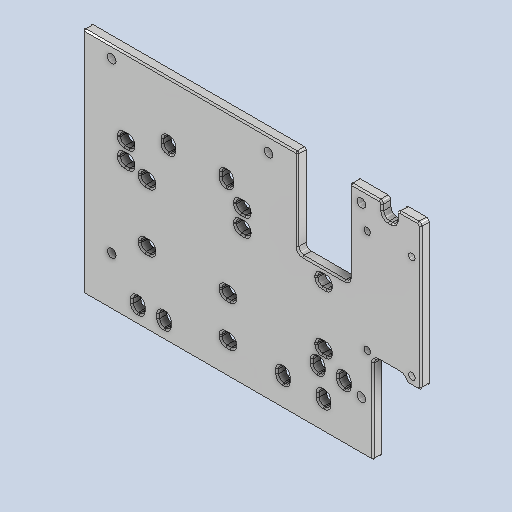
# Autodesk Inventor part: Cable_Fastener_WaveRunner
Saved by Autodesk Inventor 2022 (Build 260153000, 153)
## iProperties
Created: 2020-06-16
Part Number: Cable_Fastener_WaveRunner
Material: Generic
Document SubType Name: Modeling
Designer: Viktor Lindström
Density: 1 g/cm^3
Appearance: Default
Author: Viktor Lindström
Autodesk Inventor part; units mm, degrees
ref_plane "YZ Plane" through (0, 0, 0) normal (1, 0, 0) x (0, 1, 0)
ref_plane "XZ Plane" through (0, 0, 0) normal (0, 1, 0) x (-1, 0, 0)
ref_plane "XY Plane" through (0, 0, 0) normal (0, 0, 1) x (1, 0, 0)
sketch "Sketch1" plane through (0, 0, 0) normal (0, 0, 1) x (1, 0, 0)
  line L0 (-50, -39.5) -> (50, -39.5)
  line L1 (50, -39.5) -> (50, 39.5)
  line L2 (50, 39.5) -> (-50, 39.5)
  line L3 (-50, 39.5) -> (-50, -39.5)
  line L4 (-50, -39.5) -> (50, 39.5) construction
  line L5 (50, -39.5) -> (-50, 39.5) construction
  point P0 (0, 0)
  dimension "d0" = 100
  dimension "d1" = 79
  constraints: 12 end point, 2 midpoint, 2 parallel, 1 horizontal, 1 perpendicular
  measures "d0" distance of L1.end L2.end
  measures "d1" distance of L0.end L1.end
extrude "Extrusion1" add sketch "Sketch1" along normal blind 3
sketch "Sketch2" plane through (0, 0, 3) normal (0, 0, 1) x (1, 0, 0)
  circle A0 centre (-40, 35.5) radius 1.5
  circle A1 centre (46, 35.5) radius 1.5
  line L0 (50, 39.5) -> (-50, 39.5) projected
  line L1 (50, -39.5) -> (50, 39.5) projected
  line L2 (-73.7236, 6.5) -> (70.0965, 6.5) construction
  circle A2 centre (-40, -22.5) radius 1.5
  circle A3 centre (46, -22.5) radius 1.5
  point P0 (0, 0)
  dimension "d4" = 3
  dimension "d5" = 3
  dimension "d6" = 86
  dimension "d7" = 4
  dimension "d8" = 4
  dimension "d9" = 4
  dimension "d10" = 33
  constraints: 4 centre point, 2 end point, 2 symmetric about line, 1 horizontal, 2 other
  measures "d4" diameter of A0
  measures "d5" diameter of A1
  measures "d6" distance of A1.centre A0.centre
  measures "d7" distance from line of L0 A1.centre
  measures "d8" distance from line of L0 A0.centre
  measures "d9" distance from line of L1 A1.centre
  measures "d10" distance between parallel lines of L0 L2
extrude "Extrusion2" cut sketch "Sketch2" against normal through all
fillet "Fillet1" radius 0.6 3 edges at (-50, 39.5, 1.5) (-50, -39.5, 1.5) (50, -39.5, 1.5)
sketch "Sketch3" plane through (0, 0, 3) normal (0, 0, 1) x (1, 0, 0)
  line L0 (31, -32) -> (35, -32)
  line L1 (35, -32) -> (35, -27)
  line L2 (35, -27) -> (31, -27)
  line L3 (31, -27) -> (31, -32)
  line L4 (31, -32) -> (35, -27) construction
  line L5 (35, -32) -> (31, -27) construction
  line L6 (21, -27) -> (17, -27)
  line L7 (17, -27) -> (17, -32)
  line L8 (17, -32) -> (21, -32)
  line L9 (21, -32) -> (21, -27)
  line L10 (21, -27) -> (17, -32) construction
  line L11 (17, -27) -> (21, -32) construction
  line L12 (-2.5, -30.5) -> (2.5, -30.5)
  line L13 (2.5, -30.5) -> (2.5, -26.5)
  line L14 (2.5, -26.5) -> (-2.5, -26.5)
  line L15 (-2.5, -26.5) -> (-2.5, -30.5)
  line L16 (-2.5, -30.5) -> (2.5, -26.5) construction
  line L17 (2.5, -30.5) -> (-2.5, -26.5) construction
  line L18 (-2.5, -12.5) -> (2.5, -12.5)
  line L19 (2.5, -12.5) -> (2.5, -16.5)
  line L20 (2.5, -16.5) -> (-2.5, -16.5)
  line L21 (-2.5, -16.5) -> (-2.5, -12.5)
  line L22 (-2.5, -12.5) -> (2.5, -16.5) construction
  line L23 (2.5, -12.5) -> (-2.5, -16.5) construction
  line L24 (-18.5, 17) -> (-22.5, 17)
  line L25 (-22.5, 17) -> (-22.5, 22)
  line L26 (-22.5, 22) -> (-18.5, 22)
  line L27 (-18.5, 22) -> (-18.5, 17)
  line L28 (-18.5, 17) -> (-22.5, 22) construction
  line L29 (-22.5, 17) -> (-18.5, 22) construction
  line L30 (1.5, 17) -> (-2.5, 17)
  line L31 (-2.5, 17) -> (-2.5, 22)
  line L32 (-2.5, 22) -> (1.5, 22)
  line L33 (1.5, 22) -> (1.5, 17)
  line L34 (1.5, 17) -> (-2.5, 22) construction
  line L35 (-2.5, 17) -> (1.5, 22) construction
  line L36 (30.5, 3.5) -> (35.5, 3.5)
  line L37 (35.5, 3.5) -> (35.5, 7.5)
  line L38 (35.5, 7.5) -> (30.5, 7.5)
  line L39 (30.5, 7.5) -> (30.5, 3.5)
  line L40 (30.5, 3.5) -> (35.5, 7.5) construction
  line L41 (35.5, 3.5) -> (30.5, 7.5) construction
  line L42 (-30.3047, -16.5) -> (-25.3047, -16.5)
  line L43 (-25.3047, -16.5) -> (-25.3047, -12.5)
  line L44 (-25.3047, -12.5) -> (-30.3047, -12.5)
  line L45 (-30.3047, -12.5) -> (-30.3047, -16.5)
  line L46 (-30.3047, -16.5) -> (-25.3047, -12.5) construction
  line L47 (-25.3047, -16.5) -> (-30.3047, -12.5) construction
  line L48 (-25.3047, 3.5) -> (-30.3047, 3.5)
  line L49 (-30.3047, 3.5) -> (-30.3047, 7.5)
  line L50 (-30.3047, 7.5) -> (-25.3047, 7.5)
  line L51 (-25.3047, 7.5) -> (-25.3047, 3.5)
  line L52 (-25.3047, 3.5) -> (-30.3047, 7.5) construction
  line L53 (-30.3047, 3.5) -> (-25.3047, 7.5) construction
  line L54 (50, -38.9) -> (50, 39.5) projected
  line L55 (-49.4, -39.5) -> (49.4, -39.5) projected
  line L56 (50, 39.5) -> (-49.4, 39.5) projected
  line L57 (35.5, -16.5) -> (30.5, -16.5)
  line L58 (30.5, -16.5) -> (30.5, -12.5)
  line L59 (30.5, -12.5) -> (35.5, -12.5)
  line L60 (35.5, -12.5) -> (35.5, -16.5)
  line L61 (35.5, -16.5) -> (30.5, -12.5) construction
  line L62 (30.5, -16.5) -> (35.5, -12.5) construction
  line L63 (-50, 38.9) -> (-50, -38.9) projected
  point P0 (0, 0)
  point P1 (33, -29.5)
  point P2 (19, -29.5)
  point P3 (0, -28.5)
  point P4 (0, -14.5)
  point P5 (-20.5, 19.5)
  point P6 (-0.5, 19.5)
  point P7 (33, 5.5)
  point P8 (-27.8047, -14.5)
  point P9 (-27.8047, 5.5)
  point P10 (50, 38.9)
  point P11 (49.4, 39.5)
  point P12 (33, -14.5)
  dimension "d14" = 4
  dimension "d15" = 4
  dimension "d16" = 4
  dimension "d17" = 4
  dimension "d18" = 4
  dimension "d19" = 4
  dimension "d20" = 4
  dimension "d21" = 4
  dimension "d23" = 4
  dimension "d24" = 5
  dimension "d25" = 5
  dimension "d26" = 5
  dimension "d27" = 5
  dimension "d29" = 5
  dimension "d30" = 5
  dimension "d31" = 5
  dimension "d32" = 5
  dimension "d33" = 5
  dimension "d34" = 0
  dimension "d35" = 20
  dimension "d36" = 20
  dimension "d37" = 14
  dimension "d38" = 14
  dimension "d40" = 17
  dimension "d41" = 10
  dimension "d42" = 25
  dimension "d43" = 50
  dimension "d44" = 34
  dimension "d45" = 4
  dimension "d46" = 5
  dimension "d47" = 20
  dimension "d48" = 0
  dimension "d49" = 0
  dimension "d50" = 17
  dimension "d125" = 20
  dimension "d126" = 29.5
  constraints: 120 end point, 20 midpoint, 20 parallel, 10 horizontal, 10 perpendicular, 3 point on line
  measures "d14" distance of L14.end L12.start
  measures "d15" distance of L18.end L19.end
  measures "d16" distance of L44.end L42.start
  measures "d17" distance of L48.end L49.end
  measures "d18" distance of L24.start L24.end
  measures "d19" distance of L30.start L30.end
  measures "d20" distance of L6.start L6.end
  measures "d21" distance of L1.end L2.end
  measures "d23" distance of L38.end L36.start
  measures "d24" distance of L12.start L12.end
  measures "d25" distance of L19.end L20.end
  measures "d26" distance of L6.end L7.end
  measures "d27" distance of L2.end L0.start
  measures "d29" distance of L36.start L36.end
  measures "d30" distance of L32.end L30.start
  measures "d31" distance of L26.end L24.start
  measures "d32" distance of L48.start L48.end
  measures "d33" distance of L42.start L42.end
  measures "d34" vertical distance of point (33, -29.5) point (19, -29.5)
  measures "d35" distance of point (-27.805, 5.5) point (-27.805, -14.5)
  measures "d36" distance of point (-0.5, 19.5) point (-20.5, 19.5)
  measures "d37" distance of point (33, -29.5) point (19, -29.5)
  measures "d38" distance of point (0, -14.5) point (0, -28.5)
  measures "d40" distance from line of L54 point (33, -29.5)
  measures "d41" distance from line of L55 point (33, -29.5)
  measures "d42" distance from line of L55 point (0, -14.5)
  measures "d43" distance from line of L54 point (0, -28.5)
  measures "d44" distance from line of L56 point (-27.805, 5.5)
  measures "d45" distance of L57.end L58.end
  measures "d46" distance of L58.end L59.end
  measures "d47" distance of point (33, 5.5) point (33, -14.5)
  measures "d48" horizontal distance of point (33, 5.5) point (33, -14.5)
  measures "d49" vertical distance of point (33, -14.5) point (-27.805, -14.5)
  measures "d50" distance from line of L54 point (33, -14.5)
  measures "d125" distance from line of L56 point (-20.5, 19.5)
  measures "d126" distance from line of L63 point (-20.5, 19.5)
extrude "Extrusion3" cut sketch "Sketch3" against normal through all
sketch "Sketch4" plane through (0, 0, 3) normal (0, 0, 1) x (1, 0, 0)
  line L0 (-29, -36) -> (-33, -36)
  line L1 (-33, -36) -> (-33, -31)
  line L2 (-33, -31) -> (-29, -31)
  line L3 (-29, -31) -> (-29, -36)
  line L4 (-29, -36) -> (-33, -31) construction
  line L5 (-33, -36) -> (-29, -31) construction
  line L6 (-25.3047, -16.5) -> (-30.3047, -16.5) projected
  line L7 (-30.3047, -12.5) -> (-25.3047, -12.5) projected
  line L8 (-20, -36) -> (-24, -36)
  line L9 (-24, -36) -> (-24, -31)
  line L10 (-24, -31) -> (-20, -31)
  line L11 (-20, -31) -> (-20, -36)
  line L12 (-20, -36) -> (-24, -31) construction
  line L13 (-24, -36) -> (-20, -31) construction
  line L14 (-50, 38.9) -> (-50, -38.9) projected
  line L15 (-49.4, -39.5) -> (49.4, -39.5) projected
  line L16 (32.9777, -23) -> (28.9777, -23)
  line L17 (28.9777, -23) -> (28.9777, -18)
  line L18 (28.9777, -18) -> (32.9777, -18)
  line L19 (32.9777, -18) -> (32.9777, -23)
  line L20 (32.9777, -23) -> (28.9777, -18) construction
  line L21 (28.9777, -23) -> (32.9777, -18) construction
  line L22 (41.9777, -23) -> (37.9777, -23)
  line L23 (37.9777, -23) -> (37.9777, -18)
  line L24 (37.9777, -18) -> (41.9777, -18)
  line L25 (41.9777, -18) -> (41.9777, -23)
  line L26 (41.9777, -23) -> (37.9777, -18) construction
  line L27 (37.9777, -23) -> (41.9777, -18) construction
  line L28 (50, -38.9) -> (50, 39.5) projected
  line L29 (35, -27) -> (35, -32) projected
  line L30 (31, -27) -> (35, -27) projected
  point P0 (0, 0)
  point P1 (-31, -33.5)
  point P2 (-22, -33.5)
  point P3 (30.9777, -20.5)
  point P4 (39.9777, -20.5)
  point P5 (50, 38.9)
  dimension "d54" = 4
  dimension "d55" = 5
  dimension "d56" = 4
  dimension "d57" = 5
  dimension "d60" = 4
  dimension "d61" = 5
  dimension "d64" = 0
  dimension "d65" = 5
  dimension "d66" = 19
  dimension "d67" = 6
  dimension "d72" = 4
  dimension "d73" = 5
  dimension "d74" = 4
  dimension "d75" = 5
  dimension "d76" = 0
  dimension "d77" = 5
  dimension "d82" = 10.0223
  dimension "d83" = 2.0223
  dimension "d84" = 4
  constraints: 48 end point, 8 midpoint, 8 parallel, 4 horizontal, 4 perpendicular
  measures "d54" distance from line of L7 L6.end
  measures "d55" distance of L6.start L6.end
  measures "d56" distance of L0.start L0.end
  measures "d57" distance of L0.end L1.end
  measures "d60" distance of L8.start L8.end
  measures "d61" distance of L8.end L9.end
  measures "d64" vertical distance of point (-31, -33.5) point (-22, -33.5)
  measures "d65" distance between parallel lines of L3 L9
  measures "d66" distance from line of point (-31, -33.5) L14
  measures "d67" distance from line of L15 point (-31, -33.5)
  measures "d72" distance of L16.start L16.end
  measures "d73" distance of L16.end L17.end
  measures "d74" distance of L25.end L22.end
  measures "d75" distance of L22.end L24.start
  measures "d76" vertical distance of point (30.978, -20.5) point (39.978, -20.5)
  measures "d77" distance between parallel lines of L19 L23
  measures "d82" distance from line of L28 point (39.978, -20.5)
  measures "d83" distance between parallel lines of L29 L19
  measures "d84" distance between parallel lines of L30 L16
extrude "Extrusion4" cut sketch "Sketch4" against normal through all
sketch "Sketch5" plane through (0, 0, 3) normal (0, 0, 1) x (1, 0, 0)
  line L0 (-20, -31) -> (-20, -36) projected
  line L1 (-24, -31) -> (-20, -31) projected
  line L2 (-24, -36) -> (-24, -31) projected
  line L3 (-20, -36) -> (-24, -36) projected
  line L4 (-32.5, 15.5) -> (-37.5, 15.5)
  line L5 (-37.5, 15.5) -> (-37.5, 11.5)
  line L6 (-37.5, 11.5) -> (-32.5, 11.5)
  line L7 (-32.5, 11.5) -> (-32.5, 15.5)
  line L8 (-32.5, 15.5) -> (-37.5, 11.5) construction
  line L9 (-37.5, 15.5) -> (-32.5, 11.5) construction
  line L10 (-37.5, 9.5) -> (-32.5, 9.5)
  line L11 (-32.5, 9.5) -> (-32.5, 5.5)
  line L12 (-32.5, 5.5) -> (-37.5, 5.5)
  line L13 (-37.5, 5.5) -> (-37.5, 9.5)
  line L14 (-37.5, 9.5) -> (-32.5, 5.5) construction
  line L15 (-32.5, 9.5) -> (-37.5, 5.5) construction
  line L16 (50, 39.5) -> (-49.4, 39.5) projected
  line L17 (-50, 38.9) -> (-50, -38.9) projected
  line L18 (7.5, 15.5) -> (2.5, 15.5)
  line L19 (2.5, 15.5) -> (2.5, 11.5)
  line L20 (2.5, 11.5) -> (7.5, 11.5)
  line L21 (7.5, 11.5) -> (7.5, 15.5)
  line L22 (7.5, 15.5) -> (2.5, 11.5) construction
  line L23 (2.5, 15.5) -> (7.5, 11.5) construction
  line L24 (2.5, 9.5) -> (7.5, 9.5)
  line L25 (7.5, 9.5) -> (7.5, 5.5)
  line L26 (7.5, 5.5) -> (2.5, 5.5)
  line L27 (2.5, 5.5) -> (2.5, 9.5)
  line L28 (2.5, 9.5) -> (7.5, 5.5) construction
  line L29 (7.5, 9.5) -> (2.5, 5.5) construction
  line L30 (50, -38.9) -> (50, 39.5) projected
  point P0 (-35, 13.5)
  point P1 (-35, 7.5)
  point P2 (49.4, 39.5)
  point P3 (5, 13.5)
  point P4 (5, 7.5)
  point P5 (50, 38.9)
  dimension "d87" = 5
  dimension "d88" = 4
  dimension "d89" = 4
  dimension "d90" = 4
  dimension "d91" = 5
  dimension "d92" = 5
  dimension "d93" = 6
  dimension "d102" = 26
  dimension "d103" = 15
  dimension "d105" = 4
  dimension "d106" = 4
  dimension "d107" = 5
  dimension "d108" = 5
  dimension "d109" = 6
  dimension "d121" = 0
  dimension "d122" = 45
  constraints: 48 end point, 8 midpoint, 8 parallel, 4 horizontal, 4 perpendicular, 2 point on line
  measures "d87" distance of L0.start L0.end
  measures "d88" distance of L1.start L0.start
  measures "d89" distance between parallel lines of L12 L10
  measures "d90" distance of L4.end L5.end
  measures "d91" distance of L10.start L10.end
  measures "d92" distance of L5.end L6.end
  measures "d93" distance of point (-35, 7.5) point (-35, 13.5)
  measures "d102" distance from line of L16 point (-35, 13.5)
  measures "d103" distance from line of L17 point (-35, 13.5)
  measures "d105" distance between parallel lines of L26 L24
  measures "d106" distance of L18.end L19.end
  measures "d107" distance of L24.start L24.end
  measures "d108" distance of L19.end L20.end
  measures "d109" distance of point (5, 7.5) point (5, 13.5)
  measures "d121" distance between parallel lines of L4 L18
  measures "d122" distance from line of L30 point (5, 13.5)
extrude "Extrusion5" cut sketch "Sketch5" against normal through all contours L7 L6 L5 L4 | L10 L11 L12 L13 | L21 L20 L19 L18 | L24 L25 L26 L27
sketch "Sketch6" plane through (0, 0, 3) normal (0, 0, 1) x (1, 0, 0)
  line L0 (50, 39.5) -> (-49.4, 39.5) projected
  line L1 (24, 39.5) -> (42, 39.5)
  line L2 (42, 39.5) -> (42, 9.5)
  line L3 (42, 9.5) -> (24, 9.5)
  line L4 (24, 9.5) -> (24, 39.5)
  line L5 (50, -38.9) -> (50, 39.5) projected
  point P0 (0, 0)
  point P1 (49.4, 39.5)
  point P2 (50, 38.9)
  dimension "d127" = 30
  dimension "d128" = 8
  dimension "d129" = 18
  constraints: 8 end point, 2 parallel, 1 horizontal, 1 perpendicular, 1 point on line
  measures "d127" distance between parallel lines of L0 L3
  measures "d128" distance between parallel lines of L5 L2
  measures "d129" distance between parallel lines of L2 L4
extrude "Extrusion6" cut sketch "Sketch6" against normal through all
fillet "Fillet2" radius 0.6 2 edges at (24, 39.5, 1.5) (42, 39.5, 1.5)
fillet "Fillet2" radius 1.75 2 edges at (42, 9.5, 1.5) (24, 9.5, 1.5)
sketch "Sketch7" plane through (0, 0, 3) normal (0, 0, 1) x (1, 0, 0)
  circle A0 centre (-40, -22.5) radius 1.5 projected
  circle A1 centre (-40, 35.5) radius 1.5 projected
  circle A2 centre (46, -22.5) radius 1.5 projected
  circle A3 centre (46, 35.5) radius 1.5 projected
  arc A4 (42.6, 39.5) -> (42, 38.9) centre (42.6, 38.9) ccw projected
  line L0 (42, 38.9) -> (42, 11.25) projected
  line L1 (40.25, 9.5) -> (25.75, 9.5) projected
  line L2 (24, 11.25) -> (24, 38.9) projected
  arc A5 (24, 38.9) -> (23.4, 39.5) centre (23.4, 38.9) ccw projected
  line L3 (23.4, 39.5) -> (-49.4, 39.5) projected
  arc A6 (-49.4, 39.5) -> (-50, 38.9) centre (-49.4, 38.9) ccw projected
  line L4 (-50, 38.9) -> (-50, -38.9) projected
  arc A7 (-50, -38.9) -> (-49.4, -39.5) centre (-49.4, -38.9) ccw projected
  line L5 (-49.4, -39.5) -> (49.4, -39.5) projected
  arc A8 (49.4, -39.5) -> (50, -38.9) centre (49.4, -38.9) ccw projected
  line L6 (50, -38.9) -> (50, 39.5) projected
  line L7 (50, 39.5) -> (42.6, 39.5) projected
  line L8 (-30.3047, -12.5) -> (-25.3047, -12.5) projected
  line L9 (-25.3047, -12.5) -> (-25.3047, -16.5) projected
  line L10 (-25.3047, -16.5) -> (-30.3047, -16.5) projected
  line L11 (-30.3047, -16.5) -> (-30.3047, -12.5) projected
  line L12 (2.5, -12.5) -> (2.5, -16.5) projected
  line L13 (2.5, -16.5) -> (-2.5, -16.5) projected
  line L14 (-2.5, -16.5) -> (-2.5, -12.5) projected
  line L15 (-2.5, -12.5) -> (2.5, -12.5) projected
  line L16 (30.5, -16.5) -> (30.5, -12.5) projected
  line L17 (30.5, -12.5) -> (35.5, -12.5) projected
  line L18 (35.5, -12.5) -> (35.5, -16.5) projected
  line L19 (35.5, -16.5) -> (30.5, -16.5) projected
  line L20 (31, -27) -> (35, -27) projected
  line L21 (35, -27) -> (35, -32) projected
  line L22 (35, -32) -> (31, -32) projected
  line L23 (31, -32) -> (31, -27) projected
  line L24 (-2.5, 17) -> (-2.5, 22) projected
  line L25 (-2.5, 22) -> (1.5, 22) projected
  line L26 (1.5, 22) -> (1.5, 17) projected
  line L27 (1.5, 17) -> (-2.5, 17) projected
  line L28 (-30.3047, 3.5) -> (-30.3047, 7.5) projected
  line L29 (-30.3047, 7.5) -> (-25.3047, 7.5) projected
  line L30 (-25.3047, 7.5) -> (-25.3047, 3.5) projected
  line L31 (-25.3047, 3.5) -> (-30.3047, 3.5) projected
  line L32 (-2.5, -26.5) -> (2.5, -26.5) projected
  line L33 (2.5, -26.5) -> (2.5, -30.5) projected
  line L34 (2.5, -30.5) -> (-2.5, -30.5) projected
  line L35 (-2.5, -30.5) -> (-2.5, -26.5) projected
  line L36 (30.5, 7.5) -> (35.5, 7.5) projected
  line L37 (35.5, 7.5) -> (35.5, 3.5) projected
  line L38 (35.5, 3.5) -> (30.5, 3.5) projected
  line L39 (30.5, 3.5) -> (30.5, 7.5) projected
  line L40 (21, -32) -> (17, -32) projected
  line L41 (17, -32) -> (17, -27) projected
  line L42 (17, -27) -> (21, -27) projected
  line L43 (21, -27) -> (21, -32) projected
  line L44 (-22.5, 17) -> (-22.5, 22) projected
  line L45 (-22.5, 22) -> (-18.5, 22) projected
  line L46 (-18.5, 22) -> (-18.5, 17) projected
  line L47 (-18.5, 17) -> (-22.5, 17) projected
  line L48 (-24, -36) -> (-24, -31) projected
  line L49 (-24, -31) -> (-20, -31) projected
  line L50 (-20, -31) -> (-20, -36) projected
  line L51 (-20, -36) -> (-24, -36) projected
  line L52 (41.9777, -23) -> (37.9777, -23) projected
  line L53 (37.9777, -23) -> (37.9777, -18) projected
  line L54 (37.9777, -18) -> (41.9777, -18) projected
  line L55 (41.9777, -18) -> (41.9777, -23) projected
  line L56 (-33, -36) -> (-33, -31) projected
  line L57 (-33, -31) -> (-29, -31) projected
  line L58 (-29, -31) -> (-29, -36) projected
  line L59 (-29, -36) -> (-33, -36) projected
  line L60 (28.9777, -23) -> (28.9777, -18) projected
  line L61 (28.9777, -18) -> (32.9777, -18) projected
  line L62 (32.9777, -18) -> (32.9777, -23) projected
  line L63 (32.9777, -23) -> (28.9777, -23) projected
  line L64 (7.5, 11.5) -> (2.5, 11.5) projected
  line L65 (2.5, 11.5) -> (2.5, 15.5) projected
  line L66 (2.5, 15.5) -> (7.5, 15.5) projected
  line L67 (7.5, 15.5) -> (7.5, 11.5) projected
  line L68 (-37.5, 11.5) -> (-37.5, 15.5) projected
  line L69 (-37.5, 15.5) -> (-32.5, 15.5) projected
  line L70 (-32.5, 15.5) -> (-32.5, 11.5) projected
  line L71 (7.5, 9.5) -> (7.5, 5.5) projected
  line L72 (7.5, 5.5) -> (2.5, 5.5) projected
  line L73 (2.5, 5.5) -> (2.5, 9.5) projected
  line L74 (2.5, 9.5) -> (7.5, 9.5) projected
  line L75 (-32.5, 5.5) -> (-37.5, 5.5) projected
  arc A9 (40.25, 9.5) -> (42, 11.25) centre (40.25, 11.25) ccw projected
  arc A10 (24, 11.25) -> (25.75, 9.5) centre (25.75, 11.25) ccw projected
  line L76 (-32.5, 9.5) -> (-32.5, 5.5) projected
  line L77 (-37.5, 5.5) -> (-37.5, 9.5) projected
  line L78 (-37.5, 9.5) -> (-32.5, 9.5) projected
  line L79 (-32.5, 11.5) -> (-37.5, 11.5) projected
  point P0 (0, 0)
fillet "Fillet3" radius 1.75 47 edges at (-37.5, 15.5, 1.5) (-32.5, 15.5, 1.5) (-32.5, 11.5, 1.5) (-37.5, 11.5, 1.5) (-37.5, 5.5, 1.5) (-32.5, 9.5, 1.5) (-37.5, 9.5, 1.5) (-32.5, 5.5, 1.5) (-25.3047, 7.5, 1.5) (-30.3047, 7.5, 1.5) (-30.3047, 3.5, 1.5) (-25.3047, 3.5, 1.5) (-18.5, 17, 1.5) (-22.5, 22, 1.5) (-22.5, 17, 1.5) (-18.5, 22, 1.5) (-2.5, 22, 1.5) (-2.5, 17, 1.5) (1.5, 17, 1.5) (1.5, 22, 1.5) (2.5, 15.5, 1.5) (7.5, 15.5, 1.5) (7.5, 11.5, 1.5) (2.5, 11.5, 1.5) (2.5, 9.5, 1.5) (7.5, 9.5, 1.5) (2.5, 5.5, 1.5) (7.5, 5.5, 1.5) (30.5, 3.5, 1.5) (30.5, 7.5, 1.5) (35.5, 7.5, 1.5) (35.5, 3.5, 1.5) (41.9777, -23, 1.5) (41.9777, -18, 1.5) (35.5, -12.5, 1.5) (30.5, -12.5, 1.5) (28.9777, -18, 1.5) (37.9777, -18, 1.5) (37.9777, -23, 1.5) (28.9777, -23, 1.5) (30.5, -16.5, 1.5) (35.5, -16.5, 1.5) (32.9777, -23, 1.5) (35, -32, 1.5) (35, -27, 1.5) (31, -27, 1.5) (31, -32, 1.5)
fillet "Fillet4" radius 1.75 25 edges at (32.9777, -18, 1.5) (21, -27, 1.5) (21, -32, 1.5) (17, -32, 1.5) (17, -27, 1.5) (-2.5, -12.5, 1.5) (2.5, -12.5, 1.5) (2.5, -16.5, 1.5) (-2.5, -16.5, 1.5) (-2.5, -30.5, 1.5) (-2.5, -26.5, 1.5) (2.5, -26.5, 1.5) (2.5, -30.5, 1.5) (-30.3047, -16.5, 1.5) (-33, -36, 1.5) (-24, -36, 1.5) (-25.3047, -12.5, 1.5) (-29, -31, 1.5) (-20, -31, 1.5) (-30.3047, -12.5, 1.5) (-33, -31, 1.5) (-24, -31, 1.5) (-20, -36, 1.5) (-29, -36, 1.5) (-25.3047, -16.5, 1.5)
sketch "Sketch8" plane through (0, 0, 3) normal (0, 0, 1) x (1, 0, 0)
  circle A0 centre (14, 34.5) radius 1.5
  line L0 (23.4, 39.5) -> (-49.4, 39.5) projected
  line L1 (24, 11.25) -> (24, 38.9) projected
  point P0 (0, 0)
  dimension "d136" = 3
  dimension "d137" = 5
  dimension "d138" = 10
  constraints: 1 centre point
  measures "d136" diameter of A0
  measures "d137" distance from line of L0 A0.centre
  measures "d138" distance from line of L1 A0.centre
extrude "Extrusion7" cut sketch "Sketch8" against normal through all
sketch "Sketch9" plane through (0, 0, 3) normal (0, 0, 1) x (1, 0, 0)
  line L0 (50, -38.9) -> (50, 39.5) projected
  line L1 (50, -38.9) -> (50, 39.5) projected
  line L2 (50, 39.5) -> (66.4, 39.5)
  line L3 (66.4, 39.5) -> (66.4, -10.5)
  line L4 (66.4, -10.5) -> (50, -10.5)
  line L5 (50, -10.5) -> (50, 39.5)
  line L6 (42, 38.9) -> (42, 11.25) projected
  line L7 (50, 39.5) -> (42.6, 39.5) projected
  point P0 (0, 0)
  point P1 (50, 38.9)
  point P2 (49.4, 39.5)
  point P3 (50, -10.5)
  dimension "d144" = 24.4
  dimension "d146" = 50
  constraints: 9 end point, 2 parallel, 1 horizontal, 1 perpendicular
  measures "d144" distance between parallel lines of L3 L6
  measures "d146" distance of L2.end L3.end
extrude "Extrusion8" add sketch "Sketch9" against normal up to surface (3 mm away)
fillet "Fillet5" radius 1 3 edges at (66.4, 39.5, 1.5) (66.4, -10.5, 1.5) (50, -10.5, 1.5)
sketch "Sketch10" plane through (0, 0, 3) normal (0, 0, 1) x (1, 0, 0)
  circle A0 centre (63.4, -7.5) radius 1.15
  circle A1 centre (63.4, 28.1) radius 1.15
  circle A2 centre (48, -7.5) radius 1.15
  circle A3 centre (48, 28.1) radius 1.15
  line L0 (45.7, -9.7) -> (65.7, -9.7) construction
  line L1 (65.7, -9.7) -> (65.7, 30.3) construction
  line L2 (65.7, 30.3) -> (45.7, 30.3) construction
  line L3 (45.7, 30.3) -> (45.7, -9.7) construction
  line L4 (48, -7.5) -> (63.4, -7.5) construction
  line L5 (63.4, -7.5) -> (63.4, 28.1) construction
  line L6 (63.4, 28.1) -> (48, 28.1) construction
  line L7 (48, 28.1) -> (48, -7.5) construction
  line L8 (55.7, -7.5) -> (55.7, 28.1) construction
  line L9 (45.7, 10.3) -> (65.7, 10.3) construction
  line L10 (51, -10.5) -> (65.4, -10.5) projected
  line L11 (42, 38.9) -> (42, 11.25) projected
  line L12 (66.4, -9.5) -> (66.4, 38.5) projected
  point P0 (0, 0)
  dimension "d150" = 20
  dimension "d151" = 13.1
  dimension "d153" = 2.3
  dimension "d154" = 2.3
  dimension "d155" = 2.3
  dimension "d156" = 2.3
  dimension "d157" = 15.4
  dimension "d160" = 10
  dimension "d161" = 17.8
  dimension "d163" = 20
  dimension "d164" = 40
  dimension "d165" = 35.6
  dimension "d166" = 3
  dimension "d167" = 6
  dimension "d168" = 3
  constraints: 20 end point, 4 centre point, 4 coincident, 4 midpoint, 4 parallel, 3 horizontal, 2 perpendicular
  measures "d150" distance between parallel lines of L1 L3
  measures "d153" diameter of A2
  measures "d154" diameter of A0
  measures "d155" diameter of A3
  measures "d156" diameter of A1
  measures "d157" distance between parallel lines of L5 L7
  measures "d160" distance between parallel lines of L8 L3
  measures "d161" distance from line of L9 A2.centre
  measures "d163" distance between parallel lines of L9 L0
  measures "d164" distance between parallel lines of L2 L0
  measures "d165" distance between parallel lines of L6 L4
  measures "d166" distance from line of L10 L4.start
  measures "d167" distance from line of L11 A3.centre
  measures "d168" distance between parallel lines of L12 L5
extrude "Extrusion9" cut sketch "Sketch10" against normal blind 10
sketch "Sketch11" plane through (0, 0, 3) normal (0, 0, 1) x (1, 0, 0)
  line L0 (51, -10.5) -> (65.4, -10.5) projected
  line L1 (61.4, -19.5) -> (50, -19.5)
  line L2 (50, -19.5) -> (50, -8.5)
  line L3 (50, -8.5) -> (61.4, -8.5)
  line L4 (61.4, -8.5) -> (61.4, -19.5)
  circle A0 centre (63.4, -7.5) radius 1.15 projected
  circle A1 centre (48, -7.5) radius 1.15 projected
  point P0 (0, 0)
  point P1 (50, -11.5)
  dimension "d171" = 2
  dimension "d172" = 9
  dimension "d174" = 13.1
  dimension "d189" = 2
  dimension "d190" = 2
  constraints: 8 end point, 2 parallel, 1 horizontal, 1 perpendicular, 1 point on line
  measures "d171" distance between parallel lines of L0 L3
  measures "d172" distance between parallel lines of L0 L1
  measures "d189" distance from line of A1.centre L2
  measures "d190" distance from line of A0.centre L4
extrude "Extrusion10" cut sketch "Sketch11" against normal blind 10 contours L1 L2 L3 L4
fillet "Fillet6" radius 2 2 edges at (61.4, -8.5, 1.5) (50, -8.5, 1.5)
fillet "Fillet6" radius 1 1 edges at (61.4, -10.5, 1.5)
sketch "Sketch12" plane through (0, 0, 3) normal (0, 0, 1) x (1, 0, 0)
  line L0 (65.4, 39.5) -> (42.6, 39.5) projected
  line L1 (53.2, 39.5) -> (58.2, 39.5)
  line L2 (58.2, 39.5) -> (58.2, 34.5)
  line L3 (58.2, 34.5) -> (53.2, 34.5)
  line L4 (53.2, 34.5) -> (53.2, 39.5)
  circle A0 centre (46, 35.5) radius 1.5 projected
  circle A1 centre (63.4, 28.1) radius 1.15 projected
  circle A2 centre (48, 28.1) radius 1.15 projected
  point P0 (0, 0)
  point P1 (58.2, 39.5)
  dimension "d180" = 5
  dimension "d182" = 5
  dimension "d185" = 15.4
  dimension "d186" = 5.2
  constraints: 8 end point, 2 parallel, 1 horizontal, 1 perpendicular, 1 point on line
  measures "d180" distance between parallel lines of L0 L3
  measures "d182" distance between parallel lines of L4 L2
  measures "d185" distance of A1.centre A2.centre
  measures "d186" distance from line of L4 A2.centre
extrude "Extrusion11" cut sketch "Sketch12" against normal through all contours L2 L3 L4 L0
fillet "Fillet7" radius 1 2 edges at (53.2, 39.5, 1.5) (58.2, 39.5, 1.5)
fillet "Fillet7" radius 2 2 edges at (53.2, 34.5, 1.5) (58.2, 34.5, 1.5)
chamfer "Chamfer1" distance 0.5 angle 45 158 edges at (-50, 0, 3) (-49.8243, -39.3243, 3) (0, -39.5, 3) (49.8243, -39.3243, 3) (50, -24.7, 3) (-49.8243, 39.3243, 3) (-13, 39.5, 3) (42.1757, 39.3243, 3) (42, 25.075, 3) (41.4874, 10.0126, 3) (33, 9.5, 3) (24.5126, 10.0126, 3) (24, 25.075, 3) (23.8243, 39.3243, 3) (-19.0126, 21.4874, 3) (-20.5, 22, 3) (-21.9874, 21.4874, 3) (-22.5, 19.5, 3) (-21.9874, 17.5126, 3) (-20.5, 17, 3) (-19.0126, 17.5126, 3) (-18.5, 19.5, 3) (-33.0126, 14.9874, 3) (-35, 15.5, 3) (-36.9874, 14.9874, 3) (-37.5, 13.5, 3) (-36.9874, 12.0126, 3) (-35, 11.5, 3) (-33.0126, 12.0126, 3) (-32.5, 13.5, 3) (-25.8172, 6.9874, 3) (-27.8047, 7.5, 3) (-29.7921, 6.9874, 3) (-30.3047, 5.5, 3) (-29.7921, 4.0126, 3) (-27.8047, 3.5, 3) (-25.8172, 4.0126, 3) (-25.3047, 5.5, 3) (-33.0126, 8.9874, 3) (-35, 9.5, 3) (-36.9874, 8.9874, 3) (-37.5, 7.5, 3) (-36.9874, 6.0126, 3) (-35, 5.5, 3) (-33.0126, 6.0126, 3) (-32.5, 7.5, 3) (-27.8047, -12.5, 3) (-25.8172, -13.0126, 3) (-25.3047, -14.5, 3) (-25.8172, -15.9874, 3) (-27.8047, -16.5, 3) (-29.7921, -15.9874, 3) (-30.3047, -14.5, 3) (-29.7921, -13.0126, 3) (-29.5126, -31.5126, 3) (-31, -31, 3) (-32.4874, -31.5126, 3) (-33, -33.5, 3) (-32.4874, -35.4874, 3) (-31, -36, 3) (-29.5126, -35.4874, 3) (-29, -33.5, 3) (-20.5126, -31.5126, 3) (-22, -31, 3) (-23.4874, -31.5126, 3) (-24, -33.5, 3) (-23.4874, -35.4874, 3) (-22, -36, 3) (-20.5126, -35.4874, 3) (-20, -33.5, 3) (0, -26.5, 3) (1.9874, -27.0126, 3) (2.5, -28.5, 3) (1.9874, -29.9874, 3) (0, -30.5, 3) (-1.9874, -29.9874, 3) (-2.5, -28.5, 3) (-1.9874, -27.0126, 3) (1.9874, -13.0126, 3) (0, -12.5, 3) (-1.9874, -13.0126, 3) (-2.5, -14.5, 3) (-1.9874, -15.9874, 3) (0, -16.5, 3) (1.9874, -15.9874, 3) (2.5, -14.5, 3) (17.5126, -27.5126, 3) (17, -29.5, 3) (17.5126, -31.4874, 3) (19, -32, 3) (20.4874, -31.4874, 3) (21, -29.5, 3) (20.4874, -27.5126, 3) (19, -27, 3) (34.4874, -27.5126, 3) (33, -27, 3) (31.5126, -27.5126, 3) (31, -29.5, 3) (31.5126, -31.4874, 3) (33, -32, 3) (34.4874, -31.4874, 3) (35, -29.5, 3) (32.4652, -18.5126, 3) (30.9777, -18, 3) (29.4903, -18.5126, 3) (28.9777, -20.5, 3) (29.4903, -22.4874, 3) (30.9777, -23, 3) (32.4652, -22.4874, 3) (32.9777, -20.5, 3) (34.9874, -13.0126, 3) (33, -12.5, 3) (31.0126, -13.0126, 3) (30.5, -14.5, 3) (31.0126, -15.9874, 3) (33, -16.5, 3) (34.9874, -15.9874, 3) (35.5, -14.5, 3) (41.4652, -18.5126, 3) (39.9777, -18, 3) (38.4903, -18.5126, 3) (37.9777, -20.5, 3) (38.4903, -22.4874, 3) (39.9777, -23, 3) (41.4652, -22.4874, 3) (41.9777, -20.5, 3) (34.9874, 6.9874, 3) (33, 7.5, 3) (31.0126, 6.9874, 3) (30.5, 5.5, 3) (31.0126, 4.0126, 3) (33, 3.5, 3) (34.9874, 4.0126, 3) (35.5, 5.5, 3) (6.9874, 8.9874, 3) (5, 9.5, 3) (3.0126, 8.9874, 3) (2.5, 7.5, 3) (3.0126, 6.0126, 3) (5, 5.5, 3) (6.9874, 6.0126, 3) (7.5, 7.5, 3) (6.9874, 14.9874, 3) (5, 15.5, 3) (3.0126, 14.9874, 3) (2.5, 13.5, 3) (3.0126, 12.0126, 3) (5, 11.5, 3) (6.9874, 12.0126, 3) (7.5, 13.5, 3) (0.9874, 21.4874, 3) (-0.5, 22, 3) (-1.9874, 21.4874, 3) (-2.5, 19.5, 3) (-1.9874, 17.5126, 3) (-0.5, 17, 3) (0.9874, 17.5126, 3) (1.5, 19.5, 3)
equation "\"d5\" = d4"
equation "\"d8\" = d7"
equation "\"d21\" = d14"
equation "\"d25\" = d24"
equation "\"d26\" = d24"
equation "\"d27\" = d26"
equation "\"d29\" = d26"
equation "\"d30\" = d26"
equation "\"d31\" = d24"
equation "\"d32\" = d24"
equation "\"d33\" = d24"
equation "\"d38\" = d37"
equation "\"d46\" = d29"
equation "\"d47\" = d36"
equation "\"d56\" = d54"
equation "\"d57\" = d55"
equation "\"d61\" = d63"
equation "\"d73\" = d79"
equation "\"d75\" = d81"
equation "\"d89\" = d88"
equation "\"d90\" = d89"
equation "\"d91\" = d87"
equation "\"d92\" = d91"
equation "\"d107\" = d117"
equation "\"d108\" = d107"
equation "\"d63\" = 5"
equation "\"d79\" = 5"
equation "\"d81\" = 5"
equation "\"d117\" = 5"
body "Solid1"
